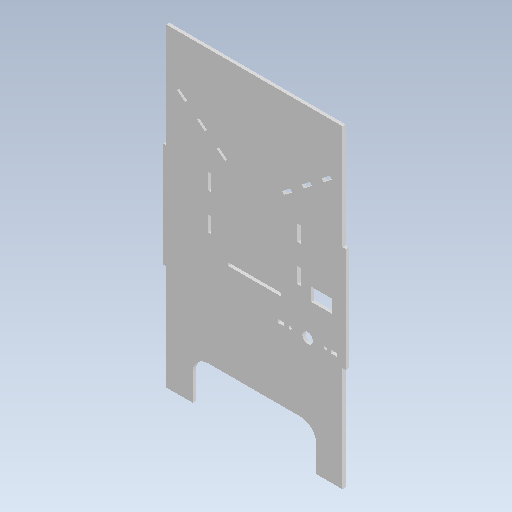
# Autodesk Inventor part: Pared_Frontal
Saved by Autodesk Inventor 2020.1 (Build 241239000, 239)
## iProperties
Created: 2019-12-08
Part Number: Pared_Frontal
Material: Generic
Document SubType Name: Modeling
Designer: Daniel
Density: 1 g/cm^3
Appearance: Default
Author: Daniel
Autodesk Inventor part; units mm, degrees
ref_plane "YZ Plane" through (0, 0, 0) normal (1, 0, 0) x (0, 1, 0)
ref_plane "XZ Plane" through (0, 0, 0) normal (0, 1, 0) x (-1, 0, 0)
ref_plane "XY Plane" through (0, 0, 0) normal (0, 0, 1) x (1, 0, 0)
sketch "Sketch1" plane through (0, 0, 0) normal (0, 0, 1) x (1, 0, 0)
  line L0 (-84, -130) -> (-84, 170) projected
  line L1 (84, -130) -> (84, 170) projected
  line L2 (-84, -130) -> (84, -130)
  line L3 (84, -130) -> (84, 170)
  line L4 (84, 170) -> (-84, 170)
  line L5 (-84, 170) -> (-84, -130)
  point P0 (0, 0)
  constraints: 8 end point, 2 parallel, 1 horizontal, 1 perpendicular
extrude "Extrusion1" add sketch "Sketch1" along normal blind 3
sketch "Sketch2" plane through (0, 0, 3) normal (0, 0, 1) x (1, 0, 0)
  line L0 (-26.2712, 87.5787) -> (-28.1182, 85.2147)
  line L1 (-28.1182, 85.2147) -> (-35.9983, 91.3713)
  line L2 (-35.9983, 91.3713) -> (-34.1513, 93.7353)
  line L3 (-34.1513, 93.7353) -> (-26.2712, 87.5787)
  line L4 (-54.9105, 106.1472) -> (-53.0636, 108.5112)
  line L5 (-53.0636, 108.5112) -> (-45.1834, 102.3546)
  line L6 (-45.1834, 102.3546) -> (-47.0304, 99.9906)
  line L7 (-47.0304, 99.9906) -> (-54.9105, 106.1472)
  line L8 (-64.0957, 117.1305) -> (-65.9427, 114.7664)
  line L9 (-65.9427, 114.7664) -> (-73.8228, 120.9231)
  line L10 (-73.8228, 120.9231) -> (-71.9758, 123.2871)
  line L11 (-71.9758, 123.2871) -> (-64.0957, 117.1305)
  point P0 (0, 0)
  constraints: 24 end point, 24 other
extrude "Extrusion2" cut sketch "Sketch2" against normal blind 10
mirror "Mirror1" about plane through (0, 0, 0) normal (1, 0, 0) of "Extrusion2"
sketch "Sketch3" plane through (0, 0, 3) normal (0, 0, 1) x (1, 0, 0)
  line L0 (44, 18) -> (41, 18)
  line L1 (41, 18) -> (41, 33)
  line L2 (41, 33) -> (44, 33)
  line L3 (44, 33) -> (44, 18)
  line L4 (44, 53) -> (41, 53)
  line L5 (41, 53) -> (41, 68)
  line L6 (41, 68) -> (44, 68)
  line L7 (44, 68) -> (44, 53)
  line L8 (-41, 18) -> (-44, 18)
  line L9 (-44, 18) -> (-44, 33)
  line L10 (-44, 33) -> (-41, 33)
  line L11 (-41, 33) -> (-41, 18)
  line L12 (-41, 53) -> (-44, 53)
  line L13 (-44, 53) -> (-44, 68)
  line L14 (-44, 68) -> (-41, 68)
  line L15 (-41, 68) -> (-41, 53)
  point P0 (0, 0)
  constraints: 32 end point, 8 horizontal, 8 vertical, 16 other
extrude "Extrusion3" cut sketch "Sketch3" against normal blind 10
sketch "Sketch4" plane through (0, 0, 3) normal (0, 0, 1) x (1, 0, 0)
  line L0 (84, -130) -> (84, 170) projected
  line L1 (84, 170) -> (87, 170)
  line L2 (87, 170) -> (87, -130)
  line L3 (87, -130) -> (84, -130)
  line L4 (84, -130) -> (84, 170)
  line L5 (-84, -130) -> (84, -130) projected
  line L6 (0, 0) -> (0, -130) construction
  line L7 (-84, -130) -> (-84, 170)
  line L8 (-84, 170) -> (-87, 170)
  line L9 (-87, 170) -> (-87, -130)
  line L10 (-87, -130) -> (-84, -130)
  line L11 (-84, -130) -> (-84, 170)
  dimension "d6" = 3
  constraints: 20 end point, 5 symmetric about line, 2 parallel, 1 collinear, 1 horizontal, 1 midpoint, 1 perpendicular
  measures "d6" distance of L0.end L1.end
extrude "Extrusion4" add sketch "Sketch4" against normal up to surface (3 mm away)
sketch "Sketch5" plane through (0, 0, 3) normal (0, 0, 1) x (1, 0, 0)
  line L0 (-87, 170) -> (-84, 170)
  line L1 (-84, 170) -> (-84, 70)
  line L2 (-84, 70) -> (-87, 70)
  line L3 (-87, 70) -> (-87, 170)
  line L4 (-84, -130) -> (-87, -130)
  line L5 (-87, -130) -> (-87, -30)
  line L6 (-87, -30) -> (-84, -30)
  line L7 (-84, -30) -> (-84, -130)
  line L8 (84, 170) -> (87, 170)
  line L9 (87, 170) -> (87, 70)
  line L10 (87, 70) -> (84, 70)
  line L11 (84, 70) -> (84, 170)
  line L12 (87, -130) -> (84, -130)
  line L13 (84, -130) -> (84, -30)
  line L14 (84, -30) -> (87, -30)
  line L15 (87, -30) -> (87, -130)
  point P0 (0, 0)
  constraints: 32 end point, 8 horizontal, 8 vertical, 16 other
extrude "Extrusion5" cut sketch "Sketch5" against normal blind 10
sketch "Sketch6" plane through (0, 0, 3) normal (0, 0, 1) x (1, 0, 0)
  line L0 (84, -130) -> (-84, -130) projected
  line L1 (-59, -130) -> (59, -130)
  line L2 (59, -130) -> (59, -90)
  line L3 (59, -90) -> (-59, -90)
  line L4 (-59, -90) -> (-59, -130)
  line L5 (84, -130) -> (84, -30) projected
  line L6 (-84, -30) -> (-84, -130) projected
  point P0 (0, 0)
  dimension "d11" = 40
  dimension "d12" = 25
  dimension "d13" = 25
  constraints: 8 end point, 2 parallel, 1 horizontal, 1 perpendicular, 1 point on line
  measures "d11" distance of L1.end L2.end
  measures "d12" distance between parallel lines of L5 L2
  measures "d13" distance between parallel lines of L6 L4
extrude "Extrusion6" cut sketch "Sketch6" against normal blind 10
fillet "Fillet1" radius 15 2 edges at (-59, -90, 1.5) (59, -90, 1.5)
sketch "Sketch8" plane through (0, 0, 3) normal (0, 0, 1) x (1, 0, 0)
  line L0 (73, -23.2) -> (73, -20)
  line L1 (73, -20) -> (79, -20)
  line L2 (79, -20) -> (79, -23.2)
  line L3 (79, -23.2) -> (73, -23.2)
  line L4 (22.5, -23.2) -> (22.5, -20)
  line L5 (22.5, -20) -> (28.5, -20)
  line L6 (28.5, -20) -> (28.5, -23.2)
  line L7 (28.5, -23.2) -> (22.5, -23.2)
  line L8 (32.5, -23.2) -> (35.5, -23.2) projected
  line L9 (35.5, -23.2) -> (35.5, -20) projected
  line L10 (32.5, -20) -> (35.5, -20) projected
  line L11 (32.5, -23.2) -> (32.5, -20) projected
  line L12 (66, -23.2) -> (69, -23.2) projected
  line L13 (69, -23.2) -> (69, -20) projected
  line L14 (66, -20) -> (69, -20) projected
  line L15 (66, -23.2) -> (66, -20) projected
  line L16 (32.5, -20) -> (35.5, -23.2) construction
  line L17 (69, -23.2) -> (66, -20) construction
  circle A0 centre (67.5, -21.6) radius 1.5
  circle A1 centre (34, -21.6) radius 1.5
  point P0 (0, 0)
  dimension "d33" = 3
  dimension "d34" = 3
  constraints: 20 end point, 4 horizontal, 4 vertical, 2 centre point, 2 midpoint, 1 parallel, 8 other
  measures "d33" diameter of A1
  measures "d34" diameter of A0
extrude "Extrusion8" cut sketch "Sketch8" against normal blind 10 contours L0 L1 L2 L3 | L4 L5 L6 L7 | A1 | A0
sketch "Sketch7" plane through (0, 0, 3) normal (0, 0, 1) x (1, 0, 0)
  line L0 (44, 33) -> (44, 18) projected
  line L1 (44, 18) -> (41, 18) projected
  line L2 (54.25, 10) -> (73.75, 10)
  line L3 (73.75, 10) -> (73.75, 22.55)
  line L4 (73.75, 22.55) -> (54.25, 22.55)
  line L5 (54.25, 22.55) -> (54.25, 10)
  line L6 (54.25, 10) -> (73.75, 22.55) construction
  line L7 (73.75, 10) -> (54.25, 22.55) construction
  line L8 (64, 19.1981) -> (64, 44.4042) construction
  line L9 (87, -30) -> (87, 70) construction
  line L10 (84, -130) -> (84, -30) projected
  line L11 (44, 18) -> (44, 33) construction
  line L12 (44, 19.1981) -> (84, 19.1981) construction
  circle A0 centre (50.75, -21.6) radius 5
  line L13 (28.5, -20) -> (28.5, -23.2) construction
  line L14 (73, -23.2) -> (73, -20) construction
  line L15 (28.5, -23.2) -> (28.5, -20) construction
  line L16 (28.5, -21.6) -> (73, -21.6) construction
  point P0 (0, 0)
  point P1 (64, 16.275)
  point P2 (64, 16.275)
  dimension "d23" = 12.55
  dimension "d24" = 19.5
  dimension "d29" = 8
  dimension "d30" = 10
  constraints: 18 end point, 9 midpoint, 3 point on line, 2 horizontal, 2 parallel, 2 perpendicular, 1 centre point, 1 vertical, 1 other
  measures "d23" distance of L2.end L3.end
  measures "d24" distance of L3.end L4.end
  measures "d29" distance between parallel lines of L1 L2
  measures "d30" diameter of A0
extrude "Extrusion7" cut sketch "Sketch7" against normal blind 10
sketch "Sketch9" plane through (0, 0, 3) normal (0, 0, 1) x (1, 0, 0)
  line L0 (25, 3) -> (25, 0)
  line L1 (25, 0) -> (-25, 0)
  line L2 (-25, 0) -> (-25, 3)
  line L3 (-25, 3) -> (25, 3)
  point P0 (0, 0)
  constraints: 8 end point, 2 horizontal, 2 vertical, 4 other
extrude "Extrusion9" cut sketch "Sketch9" against normal blind 10
body "Solid1"
